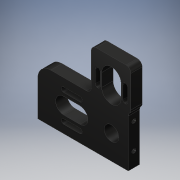
# Autodesk Inventor part: SupportMoteur
Saved by Autodesk Inventor 2019 (Build 230136000, 136)
## iProperties
Created: 2019-07-29
Part Number: SupportMoteur
Material: Plastique ABS
Document SubType Name: Modeling
Designer: Sébastien DI MERCURIO
Density: 1.06 g/cm^3
Appearance: Lustré - Noir
Mass: 23.8924 g
Surface Area: 80.29 cm^2
Volume: 22.54 cm^3
Author: Sébastien DI MERCURIO
Autodesk Inventor part; units mm, degrees
ref_plane "YZ Plane" through (0, 0, 0) normal (1, 0, 0) x (0, 1, 0)
ref_plane "XZ Plane" through (0, 0, 0) normal (0, 1, 0) x (-1, 0, 0)
ref_plane "XY Plane" through (0, 0, 0) normal (0, 0, 1) x (1, 0, 0)
sketch "Esquisse2" plane through (0, 0, 0) normal (0, 0, 1) x (1, 0, 0)
  line L0 (0, 56) -> (57.5, 56)
  line L1 (57.5, 56) -> (57.5, 0)
  line L2 (57.5, 0) -> (0, 0)
  line L3 (0, 0) -> (0, 56)
  dimension "d0" = 57.5
  dimension "d1" = 56
  constraints: 8 end point, 2 parallel, 1 coincident, 1 horizontal, 1 perpendicular
  measures "d0" distance of L0.start L0.end
  measures "d1" distance of L2.end L0.start
extrude "Extrusion1" add sketch "Esquisse2" along normal blind 7
sketch "Esquisse3" plane through (0, 0, 7) normal (0, 0, 1) x (1, 0, 0)
  line L0 (57.5, 56) -> (0, 56) projected
  line L1 (0, 56) -> (33, 56)
  line L2 (33, 56) -> (33, 30)
  line L3 (33, 30) -> (0, 30)
  line L4 (0, 30) -> (0, 56)
  line L5 (0, 0) -> (57.5, 0) projected
  line L6 (57.5, 0) -> (57.5, 56) projected
  dimension "d5" = 30
  dimension "d6" = 24.5
  constraints: 8 end point, 2 parallel, 1 horizontal, 1 perpendicular
  measures "d5" distance between parallel lines of L5 L3
  measures "d6" distance between parallel lines of L6 L2
extrude "Extrusion2" cut sketch "Esquisse3" against normal through all
sketch "Esquisse4" plane through (0, 0, 7) normal (0, 0, 1) x (1, 0, 0)
  circle A0 centre (45.5, 15) radius 4.5
  line L0 (16, 15) -> (26, 15) construction
  line L1 (16, 10) -> (26, 10)
  line L2 (26, 20) -> (16, 20)
  arc A1 (16, 20) -> (16, 10) centre (16, 15) ccw
  arc A2 (26, 10) -> (26, 20) centre (26, 15) ccw
  line L3 (16, 23.5) -> (26, 23.5) construction
  line L4 (16, 22) -> (26, 22)
  line L5 (26, 25) -> (16, 25)
  arc A3 (16, 25) -> (16, 22) centre (16, 23.5) ccw
  arc A4 (26, 22) -> (26, 25) centre (26, 23.5) ccw
  line L6 (16, 6.5) -> (26, 6.5) construction
  line L7 (16, 5) -> (26, 5)
  line L8 (26, 8) -> (16, 8)
  arc A5 (16, 8) -> (16, 5) centre (16, 6.5) ccw
  arc A6 (26, 5) -> (26, 8) centre (26, 6.5) ccw
  line L9 (45.5, 44.5) -> (45.5, 36.5) construction
  line L10 (51.5, 44.5) -> (51.5, 36.5)
  line L11 (39.5, 36.5) -> (39.5, 44.5)
  arc A7 (51.5, 44.5) -> (39.5, 44.5) centre (45.5, 44.5) ccw
  arc A8 (39.5, 36.5) -> (51.5, 36.5) centre (45.5, 36.5) ccw
  line L12 (37, 44.5) -> (37, 36.5) construction
  line L13 (38.5, 44.5) -> (38.5, 36.5)
  line L14 (35.5, 36.5) -> (35.5, 44.5)
  arc A9 (38.5, 44.5) -> (35.5, 44.5) centre (37, 44.5) ccw
  arc A10 (35.5, 36.5) -> (38.5, 36.5) centre (37, 36.5) ccw
  line L15 (54, 44.5) -> (54, 36.5) construction
  line L16 (52.5, 44.5) -> (52.5, 36.5)
  line L17 (55.5, 36.5) -> (55.5, 44.5)
  arc A11 (55.5, 44.5) -> (52.5, 44.5) centre (54, 44.5) ccw
  arc A12 (52.5, 36.5) -> (55.5, 36.5) centre (54, 36.5) ccw
  line L18 (0, 0) -> (57.5, 0) projected
  line L19 (57.5, 0) -> (57.5, 56) projected
  line L20 (33, 56) -> (33, 30) projected
  line L21 (57.5, 56) -> (33, 56) projected
  line L22 (0, 30) -> (0, 0) projected
  point P0 (21, 15)
  point P1 (21, 23.5)
  point P2 (21, 6.5)
  point P3 (45.5, 40.5)
  point P4 (37, 40.5)
  point P5 (54, 40.5)
  dimension "d9" = 12
  dimension "d10" = 3
  dimension "d11" = 3
  dimension "d12" = 3
  dimension "d13" = 3
  dimension "d14" = 10
  dimension "d15" = 9
  dimension "d19" = 13
  dimension "d20" = 13
  dimension "d21" = 20
  dimension "d22" = 20
  dimension "d23" = 11
  dimension "d24" = 11
  dimension "d25" = 1
  dimension "d26" = 1
  dimension "d27" = 2
  dimension "d28" = 2
  dimension "d30" = 15
  dimension "d31" = 12
  dimension "d32" = 5
  dimension "d33" = 2.5
  dimension "d34" = 5.5
  dimension "d37" = 16
  dimension "d38" = 0
  dimension "d39" = 0
  dimension "d40" = 0
  dimension "d41" = 0
  constraints: 48 end point, 24 point on circle, 24 tangent, 13 centre point, 9 parallel, 6 midpoint, 1 horizontal, 1 perpendicular, 1 vertical
  measures "d9" distance between parallel lines of L10 L11
  measures "d10" distance between parallel lines of L13 L14
  measures "d11" distance between parallel lines of L17 L16
  measures "d12" distance between parallel lines of L4 L5
  measures "d13" distance between parallel lines of L7 L8
  measures "d14" distance between parallel lines of L1 L2
  measures "d15" diameter of A0
  measures "d25" distance between parallel lines of L13 L11
  measures "d26" distance between parallel lines of L10 L16
  measures "d27" distance between parallel lines of L2 L4
  measures "d28" distance between parallel lines of L1 L8
  measures "d30" distance from line of L18 A0.centre
  measures "d31" distance from line of L19 A0.centre
  measures "d32" distance between parallel lines of L18 L7
  measures "d33" distance between parallel lines of L20 L14
  measures "d34" distance edge to line of A7 L21
  measures "d37" distance from line of L22 L0.start
  measures "d38" horizontal distance of point (21, 15) point (21, 23.5)
  measures "d39" horizontal distance of point (21, 6.5) point (21, 15)
  measures "d40" vertical distance of point (45.5, 40.5) point (37, 40.5)
  measures "d41" vertical distance of point (45.5, 40.5) point (54, 40.5)
extrude "Extrusion3" cut sketch "Esquisse4" against normal through all
fillet "Congé1" radius 8 1 edges at (0, 30, 3.5)
fillet "Congé2" radius 3 3 edges at (33, 56, 3.5) (57.5, 56, 3.5) (33, 30, 3.5)
sketch "Esquisse5" plane through (0, 0, 7) normal (0, 0, 1) x (1, 0, 0)
  line L0 (57.5, 32) -> (55.9, 32)
  line L1 (55.9, 32) -> (55.9, 0)
  line L2 (55.9, 0) -> (57.5, 0)
  line L3 (57.5, 0) -> (57.5, 32)
  line L4 (57.5, 0) -> (57.5, 53) projected
  line L5 (0, 0) -> (57.5, 0) projected
  dimension "d46" = 1.6
  dimension "d47" = 32
  constraints: 8 end point, 2 collinear, 2 parallel, 1 horizontal, 1 perpendicular
  measures "d46" distance of L0.start L0.end
  measures "d47" distance of L2.end L0.start
extrude "Extrusion4" cut sketch "Esquisse5" against normal through all
fillet "Congé3" radius 3 2 edges at (55.9, 32, 3.5) (57.5, 32, 3.5)
sketch "Esquisse6" plane through (55.9, 0, 7) normal (1, 0, 0) x (0, 0, -1)
  circle A0 centre (3.5, 9) radius 1.25
  circle A1 centre (3.5, 25) radius 1.25
  line L0 (7, 29.3467) -> (7, 0) projected
  line L1 (7, 0) -> (0, 0) projected
  dimension "d51" = 2.5
  dimension "d52" = 2.5
  dimension "d53" = 3.5
  dimension "d54" = 3.5
  dimension "d55" = 16
  dimension "d56" = 9
  constraints: 2 centre point
  measures "d51" diameter of A1
  measures "d52" diameter of A0
  measures "d53" horizontal distance of A0.centre L0.end
  measures "d54" distance from line of L0 A1.centre
  measures "d55" distance of A1.centre A0.centre
  measures "d56" distance from line of L1 A0.centre
extrude "Extrusion5" cut sketch "Esquisse6" against normal blind 5
sketch "Esquisse7" plane through (0, 0, 0) normal (0, -1, 0) x (1, 0, 0)
  circle A0 centre (8.9, 3.5) radius 1.25
  circle A1 centre (31.9, 3.5) radius 1.25
  circle A2 centre (42.9, 3.5) radius 1.25
  line L0 (55.9, 0) -> (0, 0) projected
  line L1 (57.5, 0) -> (57.5, 7) projected
  line L2 (0, 0) -> (0, 7) projected
  line L3 (55.9, 0) -> (55.9, 7) projected
  dimension "d59" = 2.5
  dimension "d60" = 2.5
  dimension "d61" = 2.5
  dimension "d62" = 3.5
  dimension "d63" = 3.5
  dimension "d64" = 3.5
  dimension "d65" = 11
  dimension "d70" = 13
  dimension "d71" = 23
  constraints: 3 centre point
  measures "d59" diameter of A2
  measures "d60" diameter of A1
  measures "d61" diameter of A0
  measures "d62" distance from line of L0 A0.centre
  measures "d63" distance from line of L0 A1.centre
  measures "d64" distance from line of L0 A2.centre
  measures "d65" distance of A2.centre A1.centre
  measures "d70" distance from line of L3 A2.centre
  measures "d71" distance of A0.centre A1.centre
extrude "Extrusion6" cut sketch "Esquisse7" against normal blind 5
equation "\"d52\" = d51"
equation "\"d54\" = d53"
equation "\"d60\" = d59"
equation "\"d61\" = d59"
equation "\"d63\" = d62"
equation "\"d64\" = d62"
